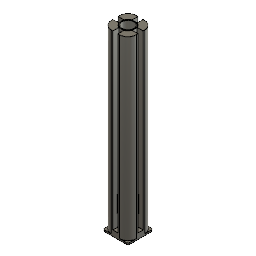
rodv4 (Autodesk Fusion 360 design; units mm, degrees)
Autodesk Fusion 360 part; units mm, degrees
sketch "Sketch1" plane through (0, 0, 0) normal (0, 1, 0) x (1, 0, 0)
  circle A0 centre (0, 0) radius 4
  circle A1 centre (0, 0) radius 4.2
  line L0 (7.5, 7.5) -> (-7.5, 7.5)
  line L1 (-7.5, 7.5) -> (-7.5, -7.5)
  line L2 (-7.5, -7.5) -> (7.5, -7.5)
  line L3 (7.5, -7.5) -> (7.5, 7.5)
  line L4 (7.5, 7.5) -> (-7.5, -7.5) construction
  line L5 (-7.5, 7.5) -> (7.5, -7.5) construction
  dimension "d1" = 8
  dimension "d2" = 8.4
  dimension "d3" = 15
  dimension "d4" = 15
  measures "d1" diameter of A0
  measures "d2" diameter of A1
extrude "Extrude1" add sketch "Sketch1" along normal blind 3 makes body 1 at (3.995, 2, 0.1994) makes body 2 at (-0.1046, 0, 6.3961)
sketch "Sketch2" plane through (0, 3, 0) normal (0, 1, 0) x (-1, 0, 0)
  circle A0 centre (0, 0) radius 4
  line L0 (-1.5, -7.5) -> (1.5, -7.5)
  line L1 (1.5, -7.5) -> (1.5, 7.5)
  line L2 (1.5, 7.5) -> (-1.5, 7.5)
  line L3 (-1.5, 7.5) -> (-1.5, -7.5)
  line L4 (-1.5, -7.5) -> (1.5, 7.5) construction
  line L5 (1.5, -7.5) -> (-1.5, 7.5) construction
  line L6 (-7.5, -1.5) -> (7.5, -1.5)
  line L7 (7.5, -1.5) -> (7.5, 1.5)
  line L8 (7.5, 1.5) -> (-7.5, 1.5)
  line L9 (-7.5, 1.5) -> (-7.5, -1.5)
  line L10 (-7.5, -1.5) -> (7.5, 1.5) construction
  line L11 (7.5, -1.5) -> (-7.5, 1.5) construction
  line L12 (-7.5, 7.5) -> (-7.5, -7.5)
  dimension "d7" = 3
  dimension "d8" = 3
extrude "Extrude2" cut sketch "Sketch2" against normal blind 0.5 contours A0 L6 L7 L8 | A0 L1 L2 L3 | A0 L0 L1 L3 | A0 L6 L8 L9 L12 bodies 2
extrude "Extrude3" add 5 faces at (3.8421, 3, 6.1185) (-6.1185, 3, 3.8421) (-0.9774, 3, -0.9069) (-6.1185, 3, -3.8421) (3.8421, 3, -6.1185) along direction (0, 1, 0) blind 7 on bodies 1 2 bodies 2 1
sketch "Sketch3" plane through (0, 10, 0) normal (0, 1, 0) x (-1, 0, 0)
  circle A0 centre (0, 0) radius 4
  line L0 (-7.5, -7.5) -> (7.5, -7.5)
  line L1 (7.5, -7.5) -> (7.5, 7.5)
  line L2 (7.5, 7.5) -> (-7.5, 7.5)
  line L3 (-7.5, 7.5) -> (-7.5, -7.5)
  line L4 (-7.5, -7.5) -> (7.5, 7.5) construction
  line L5 (7.5, -7.5) -> (-7.5, 7.5) construction
  circle A1 centre (0, 0) radius 5.1
  dimension "d15" = 10.2
  measures "d15" diameter of A1
extrude "Extrude4" cut 4 faces at (3.8421, 10, -6.1185) (-6.1185, 10, -3.8421) (-6.1185, 10, 3.8421) (3.8421, 10, 6.1185) along direction (0, -1, 0) blind 0.4 on bodies 2 bodies 2
extrude "Extrude5" add sketch "Sketch3" against normal blind 0.4 contours L0 L1 L2 L3 bodies 2
sketch "Sketch4" plane through (0, 10, 0) normal (0, 1, 0) x (-1, 0, 0)
  circle A0 centre (0, 0) radius 4
  line L0 (-1.5, -7.5) -> (1.5, -7.5)
  line L1 (1.5, -7.5) -> (1.5, 7.5)
  line L2 (1.5, 7.5) -> (-1.5, 7.5)
  line L3 (-1.5, 7.5) -> (-1.5, -7.5)
  line L4 (-1.5, -7.5) -> (1.5, 7.5) construction
  line L5 (1.5, -7.5) -> (-1.5, 7.5) construction
  line L6 (-7.5, -1.5) -> (7.5, -1.5)
  line L7 (7.5, -1.5) -> (7.5, 1.5)
  line L8 (7.5, 1.5) -> (-7.5, 1.5)
  line L9 (-7.5, 1.5) -> (-7.5, -1.5)
  line L10 (-7.5, -1.5) -> (7.5, 1.5) construction
  line L11 (7.5, -1.5) -> (-7.5, 1.5) construction
extrude "Extrude6" cut sketch "Sketch4" against normal blind 0.4 contours A0 L6 L7 L8 | A0 L1 L2 L3 | A0 L0 L1 L3 | A0 L6 L8 L9 bodies 2
sketch "Sketch5" plane through (0, 10, 0) normal (0, 1, 0) x (-1, 0, 0)
  circle A0 centre (0, 0) radius 4
  circle A1 centre (0, 0) radius 4.9
  dimension "d20" = 9.8
  measures "d20" diameter of A1
extrude "Extrude7" add sketch "Sketch5" along normal blind 9 contours A0 | A1 bodies 1
extrude "Extrude8" add 4 faces at (6.425, 10, 3.927) (-3.927, 10, 6.425) (-3.927, 10, -6.425) (6.425, 10, -3.927) along direction (0, 1, 0) blind 9 on bodies 2 bodies 2
extrude "Extrude9" add 4 faces at (6.425, 19, -3.927) (6.425, 19, 3.927) (-3.927, 19, 6.425) (-3.927, 19, -6.425) along direction (0, 1, 0) blind 0.4 on bodies 2 bodies 2
sketch "Sketch6" plane through (0, 19, 0) normal (0, 1, 0) x (-1, 0, 0)
  circle A0 centre (0, 0) radius 4.9
  circle A1 centre (0, 0) radius 4
  dimension "d27" = 8
  measures "d27" diameter of A1
extrude "Extrude10" add sketch "Sketch6" along normal blind 0.4 contours A1 bodies 1
sketch "Sketch7" plane through (0, 19.4, 0) normal (0, 1, 0) x (-1, 0, 0)
  circle A0 centre (0, 0) radius 4
  line L0 (-7.5, -7.5) -> (7.5, -7.5)
  line L1 (7.5, -7.5) -> (7.5, 7.5)
  line L2 (7.5, 7.5) -> (-7.5, 7.5)
  line L3 (-7.5, 7.5) -> (-7.5, -7.5)
  line L4 (-7.5, -7.5) -> (7.5, 7.5) construction
  line L5 (7.5, -7.5) -> (-7.5, 7.5) construction
  circle A1 centre (0, 0) radius 4.2
  line L6 (-1.5, -7.5) -> (1.5, -7.5)
  line L7 (1.5, -7.5) -> (1.5, 7.5)
  line L8 (1.5, 7.5) -> (-1.5, 7.5)
  line L9 (-1.5, 7.5) -> (-1.5, -7.5)
  line L10 (-1.5, -7.5) -> (1.5, 7.5) construction
  line L11 (1.5, -7.5) -> (-1.5, 7.5) construction
  line L12 (-7.5, -1.5) -> (7.5, -1.5)
  line L13 (7.5, -1.5) -> (7.5, 1.5)
  line L14 (7.5, 1.5) -> (-7.5, 1.5)
  line L15 (-7.5, 1.5) -> (-7.5, -1.5)
  line L16 (-7.5, -1.5) -> (7.5, 1.5) construction
  line L17 (7.5, -1.5) -> (-7.5, 1.5) construction
  dimension "d30" = 8.4
  measures "d30" diameter of A1
extrude "Extrude11" add sketch "Sketch7" along normal blind 0.6 contours L1 L2 A1 L7 L14 | L0 L1 A1 L7 L12 | L2 L3 A1 L9 L14 | L0 L3 A1 L9 L12 bodies 2
extrude "Extrude12" add 1 faces at (1.2456, 19.4, 0.0132) along direction (0, 1, 0) blind 0.6 on bodies 1 bodies 1
extrude "Extrude13" add 5 faces at (3.8421, 20, 6.1185) (1.2456, 20, 0.0132) (-3.8421, 20, 6.1185) (-3.8421, 20, -6.1185) (3.8421, 20, -6.1185) along direction (0, 1, 0) blind 85 on bodies 1 2 bodies 2 1
fillet "Fillet1" radius 5 1 edges at (-7.5, 52.5, -7.5) on bodies 2
fillet "Fillet2" radius 5 1 edges at (-7.5, 52.5, 7.5) on bodies 2
fillet "Fillet3" radius 5 1 edges at (7.5, 52.5, 7.5) on bodies 2
fillet "Fillet4" radius 5 1 edges at (7.5, 52.5, -7.5) on bodies 2
sketch "Sketch8" plane through (0, 105, 0) normal (0, 1, 0) x (-1, 0, 0)
  circle A0 centre (0, 0) radius 4
  circle A1 centre (0, 0) radius 3.5
  dimension "d41" = 7
  measures "d41" diameter of A1
extrude "Extrude14" cut sketch "Sketch8" against normal blind 6 contours A1 bodies 1
sketch "Sketch9" plane through (0, 0, 0) normal (0, -1, 0) x (1, 0, 0)
  circle A0 centre (0, 0) radius 4
extrude "Extrude15" cut sketch "Sketch9" against normal blind 0.2 bodies 1
chamfer "Chamfer1" distance 0.4 angle 45 1 edges at (-3.7293, 0.2, 1.4465) on bodies 1
sketch "Sketch10" plane through (0, 0.2, 0) normal (0, -1, 0) x (1, 0, 0)
  circle A0 centre (0, 0) radius 3.6
  circle A1 centre (0, 0) radius 0.4
  dimension "d47" = 0.8
  measures "d47" diameter of A1
extrude "Extrude16" add sketch "Sketch10" along normal blind 0.2 contours A1 bodies 1
sketch "Sketch11" plane through (0, 0, 0) normal (0, -1, 0) x (1, 0, 0)
  circle A0 centre (0, 0) radius 0.4
  line L0 (7.5, 7.5) -> (-7.5, 7.5)
  line L1 (-7.5, 7.5) -> (-7.5, -7.5)
  line L2 (-7.5, -7.5) -> (7.5, -7.5)
  line L3 (7.5, -7.5) -> (7.5, 7.5)
  line L4 (7.5, 7.5) -> (-7.5, -7.5) construction
  line L5 (-7.5, 7.5) -> (7.5, -7.5) construction
  dimension "d50" = 15
  dimension "d51" = 15
extrude "Extrude17" add sketch "Sketch11" along normal blind 1 bodies 2 1
extrude "Extrude18" add 1 faces at (0.2105, 0, -0.1435) along direction (0, -1, 0) blind 1 on bodies 2 bodies 2
fillet "Fillet5" radius 1 2 edges at (7.5, -0.5, 7.5) (-7.5, -0.5, 7.5) on bodies 2
fillet "Fillet6" radius 1 1 edges at (7.5, -0.5, -7.5) on bodies 2
fillet "Fillet7" radius 1 1 edges at (-7.5, -0.5, -7.5) on bodies 2
